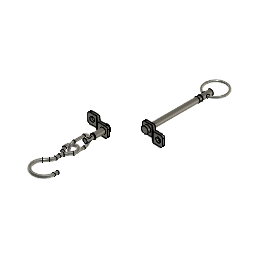
load_cell_tension_system (Autodesk Fusion 360 design; units mm, degrees)
Autodesk Fusion 360 part; units mm, degrees
note: some values were not read from the file. Chosen so that the rebuilt part matches the saved one: which face or edge a step refers to; a direction. Set by a fixed rule: which sketch regions a step uses.
sketch "Sketch1" plane through (0, 0, 0) normal (0, 0, 1) x (1, 0, 0)
  line L0 (30, -6.35) -> (-30, -6.35) construction
  line L1 (-30, -6.35) -> (-30, 6.35) construction
  line L2 (-30, 6.35) -> (30, 6.35) construction
  line L3 (30, 6.35) -> (30, -6.35) construction
  line L4 (30, -6.35) -> (-30, 6.35) construction
  line L5 (-30, -6.35) -> (30, 6.35) construction
  line L6 (-29.2721, -6.35) -> (-20, -6.35)
  line L7 (-20, -6.35) -> (-14.636, -10.8509)
  line L8 (-14.636, -10.8509) -> (-5.364, -10.8509)
  line L9 (-29.2721, -8.35) -> (-20.7279, -8.35)
  line L10 (-20.7279, -8.35) -> (-15.364, -12.8509)
  line L11 (-15.364, -12.8509) -> (-5.364, -12.8509)
  line L12 (-29.2721, -6.35) -> (-29.2721, -8.35)
  line L13 (-5.364, -10.8509) -> (-5.364, -12.8509)
  point P0 (-25, -8.35)
  point P1 (-10, -10.8509)
  dimension "d1" = 12.7
  dimension "d2" = 60
  dimension "d3" = 2
  dimension "d4" = 140
  dimension "d6" = 10
  dimension "d7" = 5
  dimension "d9" = 15
  constraint horizontal L0
  constraint perpendicular L0 L1
  constraint parallel L0 L2
  constraint parallel L1 L3
  constraint coincident L4 origin
  constraint coincident L5 origin
  constraint coincident L0 L6.start
  constraint coincident L0 L6.end
  constraint parallel L0 L8
  constraint equal L6 L8
  constraint vertical L12
  constraint vertical L13
  constraint midpoint L9 P0
  constraint midpoint L8 P1
  measures "d1" distance of L0.end L1.end
  measures "d2" distance of L0.start L0.end
  measures "d4" angle of L7 L8
  measures "d6" distance of L10.end L11.end
  measures "d7" horizontal distance of L0.end P0
  measures "d9" horizontal distance of P0 P1
extrude "Extrude1" add sketch "Sketch1" along normal mid plane 10 makes body 1
fillet "Fillet1" radius 2 4 edges at (-5.364, -11.8509, 5) (-5.364, -11.8509, -5) (-29.2721, -7.35, 5) (-29.2721, -7.35, -5) on bodies 1
sketch "Sketch2" plane through (0, -8.35, 0) normal (0, -1, 0) x (1, 0, 0)
  arc A0 (-29.2721, -3) -> (-27.2721, -5) centre (-27.2721, -3) ccw
  line L0 (-27.2721, -5) -> (-20.7279, -5)
  line L1 (-20.7279, -5) -> (-20.7279, 5)
  line L2 (-20.7279, 5) -> (-27.2721, 5)
  arc A1 (-27.2721, 5) -> (-29.2721, 3) centre (-27.2721, 3) ccw
  line L3 (-29.2721, 3) -> (-29.2721, -3)
  point P0 (-25, 0)
  point P1 (-10, 0)
hole "Hole1" at (-25, -8.35, 0) direction (0, 1, 0) diameter 4.5 depth 7 tip angle 180 bodies 1
hole "Hole2" at (-10, -8.35, 0) direction (0, -1, 0) diameter 5.5 depth 7 tip angle 180 bodies 1
mirror "Mirror1" about plane through (0, 0, 0) normal (1, 0, 0) of bodies 1 makes body 2
mirror "Mirror2" about plane through (0, 0, 0) normal (0, 1, 0) of bodies 2 makes body 3
delete_body "RemoveBody1" bodies 2
sketch "Sketch3" plane through (0, 12.8509, 0) normal (0, 1, 0) x (-1, 0, 0)
  circle A0 centre (-10, 0) radius 2.75
  arc A1 (-7.364, -5) -> (-5.364, -3) centre (-7.364, -3) ccw
  line L0 (-5.364, -3) -> (-5.364, 3)
  arc A2 (-5.364, 3) -> (-7.364, 5) centre (-7.364, 3) ccw
  line L1 (-7.364, 5) -> (-15.364, 5)
  line L2 (-15.364, 5) -> (-15.364, -5)
  line L3 (-15.364, -5) -> (-7.364, -5)
  circle A3 centre (-10, 0) radius 2.5
  dimension "d24" = 5
  constraint concentric A0 A3
  measures "d24" diameter of A3
extrude "Extrude2" add sketch "Sketch3" along normal blind 60 and the other way blind 2.1 separate body contours A3 makes body 4
sketch "Sketch4" plane through (0, 0, 0) normal (0, 0, 1) x (1, 0, 0)
  line L0 (12, 62.8509) -> (14.4908, 62.8509)
  line L1 (14.4908, 62.8509) -> (14.4908, 59.8509)
  line L2 (14.4908, 59.8509) -> (12, 59.8509)
  line L3 (12, 59.8509) -> (12, 62.8509)
  line L4 (12.5, 72.8509) -> (7.5, 72.8509)
  line L5 (10, 72.8509) -> (10, 59.2926)
  line L6 (7.5, 10.7509) -> (12.5, 10.7509)
  line L7 (12.5, 10.7509) -> (13, 10.7509)
  line L8 (10, 10.7509) -> (10, 10.2509)
  line L9 (13, 10.7509) -> (13, 10.2509)
  line L10 (13, 10.2509) -> (10, 10.2509)
  dimension "d29" = 2
  dimension "d30" = 3
  dimension "d31" = 10
  dimension "d33" = 0.5
  dimension "d35" = 0.5
  constraint horizontal L0
  constraint vertical L1
  constraint horizontal L2
  constraint vertical L3
  constraint midpoint L4 L5.start
  constraint perpendicular L4 L5
  constraint coincident L6.end L7.start
  constraint horizontal L7
  constraint midpoint L6 L8.start
  constraint vertical L8
  constraint perpendicular L7 L9
  constraint horizontal L10
  measures "d29" distance of L3 L5
  measures "d30" distance of L0.start L2.end
  measures "d31" distance of L0.start L4
  measures "d33" distance of L6.end L7.end
  measures "d35" distance of L8.end L8.start
revolve "Revolve1" cut sketch "Sketch4" angle 360 about axis through (10, 72.8509, 0) along (0, -1, 0) contours L0 L1 L2 L3 bodies 4
revolve "Revolve2" add sketch "Sketch4" angle 360 about axis through (10, 10.7509, 0) along (0, -1, 0) contours L6 L7 L8 L9 L10 bodies 4
ref_plane "WorkPlane1" through (10, 66.0717, 0) normal (-1, 0, 0) x (0, -1, 0)
sketch "Sketch5" plane through (10, 0, 0) normal (-1, 0, 0) x (0, -1, 0)
  circle A0 centre (-67.8509, 0) radius 1.5
  circle A1 centre (-67.8509, 0) radius 1
  point P0 (-72.8509, 0)
  dimension "d43" = 5
  dimension "d44" = 3
  dimension "d45" = 2
  constraint concentric A0 A1
  constraint horizontal A0.centre origin
  measures "d43" distance of A0.centre P0
  measures "d44" diameter of A0
  measures "d45" diameter of A1
extrude "Extrude3" cut sketch "Sketch5" along normal mid plane 28 contours A0 | A1 bodies 4
sketch "Sketch6" plane through (0, 0, 0) normal (0, 0, 1) x (1, 0, 0)
  circle A0 centre (10, 77.8509) radius 10
  point P0 (10, 67.8509)
  dimension "d46" = 20
  constraint coincident A0 P0
  constraint vertical A0.centre P0
  measures "d46" diameter of A0
sweep "Sweep1" add profiles "Sketch5" path "Sketch6" along A0 section 1 contours A1 separate body makes body 5
sketch "Sketch7" plane through (0, 0, 0) normal (0, 0, 1) x (1, 0, 0)
  line L0 (-7.25, -12.8509) -> (-12.75, -12.8509)
  line L1 (-10, -10.2509) -> (-10, -30.2509)
  line L2 (-10, -10.2509) -> (-7, -10.2509)
  line L3 (-7, -10.2509) -> (-7, -10.7509)
  line L4 (-7, -10.7509) -> (-7.5, -10.7509)
  line L5 (-7.5, -10.7509) -> (-7.5, -22.2509)
  line L6 (-7.5, -22.2509) -> (-8, -22.2509)
  line L7 (-8, -22.2509) -> (-8, -30.2509)
  line L8 (-8, -30.2509) -> (-10, -30.2509)
  line L9 (-7.364, -10.8509) -> (-14.636, -10.8509)
  point P0 (-10, -12.8509)
  point P1 (-10, -12.8509)
  dimension "d53" = 2.5
  dimension "d54" = 0.5
  dimension "d55" = 0.1
  dimension "d56" = 20
  dimension "d57" = 8
  dimension "d58" = 0.5
  dimension "d59" = 0.5
  constraint perpendicular L0 L1
  constraint midpoint L0 P1
  constraint coincident L1 P1
  constraint coincident P1 P0
  constraint perpendicular L1 L2
  constraint perpendicular L2 L3
  constraint perpendicular L3 L4
  constraint perpendicular L5 L6
  constraint perpendicular L0 L7
  constraint perpendicular L1 L8
  constraint vertical L5
  measures "d53" distance of L1 L5
  measures "d54" distance of L3.end L4.end
  measures "d55" distance of L4 L9
  measures "d56" distance of L1.start L1.end
  measures "d57" distance of L6.end L7.end
  measures "d58" distance of L2.end L3.end
  measures "d59" distance of L5.end L6.end
revolve "Revolve3" add sketch "Sketch7" angle 360 about axis through (-10, -10.2509, 0) along (0, -1, 0) separate body makes body 6
sketch "Sketch8" plane through (0, 0, 0) normal (0, 0, 1) x (1, 0, 0)
  circle A0 centre (-10, -26.2509) radius 1.2
  line L0 (-11.25, -26.0009) -> (-11.25, -27.0009)
  arc A1 (-11.25, -27.0009) -> (-8.75, -27.0009) centre (-10, -27.0009) ccw
  line L1 (-8.75, -27.0009) -> (-8.75, -26.0009)
  arc A2 (-8.75, -26.0009) -> (-11.25, -26.0009) centre (-10, -26.0009) ccw
  line L2 (-10, -24.7509) -> (-10, -28.2509) construction
  point P0 (-10, -12.8509)
  point P1 (-10, -30.2509)
  dimension "d62" = 2.4
  dimension "d63" = 4
  dimension "d76" = 2.5
  dimension "d77" = 3.5
  dimension "d80" = 1.5
  constraint vertical A0.centre P1
  constraint tangent L0 A1
  constraint tangent A1 L1
  constraint parallel L0 L1
  constraint tangent L1 A2
  constraint tangent L0 A2
  constraint midpoint A2 L2.start
  constraint midpoint A1 L2.end
  constraint vertical L2
  constraint vertical P1 L2.start
  measures "d62" diameter of A0
  measures "d63" distance of A0.centre P1
  measures "d76" distance of L0 L1
  measures "d77" distance of L2.start L2.end
  measures "d80" distance of A0.centre L2.start
extrude "Extrude4" cut sketch "Sketch8" along normal mid plane 6 contours A0 | L0 A1 L1 A2 bodies 6
ref_plane "WorkPlane2" through (-10, -20.2509, 0) normal (-1, 0, 0) x (0, -1, 0)
sketch "Sketch9" plane through (-10, 0, 0) normal (-1, 0, 0) x (0, -1, 0)
  line L0 (41.2509, 5) -> (31.2509, 5)
  arc A0 (31.2509, 5) -> (31.2509, -5) centre (31.2509, 0) ccw
  line L1 (31.2509, -5) -> (41.2509, -5)
  arc A1 (41.2509, -5) -> (41.2509, 5) centre (41.2509, 0) ccw
  line L2 (46.2509, 0) -> (26.2509, 0) construction
  point P0 (26.2509, 0)
  dimension "d67" = 10
  dimension "d68" = 20
  constraint tangent L0 A0
  constraint tangent A0 L1
  constraint parallel L0 L1
  constraint tangent L1 A1
  constraint tangent L0 A1
  constraint midpoint A1 L2.start
  constraint midpoint A0 P0
  constraint horizontal L2
  constraint horizontal P0 L2.end
  constraint coincident P0 L2.end
  measures "d67" distance of L0 L1
  measures "d68" distance of L2.start P0
sweep "Sweep2" add profiles "Sketch8" path "Sketch9" along A1 L0 A0 L1 section 1 contours A0 separate body makes body 7
fillet "Fillet2" radius 0.5 1 edges at (-11.8647, -22.2509, -0.7232) on bodies 6
sketch "Sketch10" plane through (-10, 0, 0) normal (-1, 0, 0) x (0, -1, 0)
  circle A0 centre (38.7509, 0) radius 1.5
  point P0 (41.2509, 0)
  dimension "d81" = 2.5
  dimension "d82" = 3
  constraint horizontal A0.centre P0
  measures "d81" horizontal distance of A0.centre P0
  measures "d82" diameter of A0
sketch "Sketch11" plane through (0, 0, 0) normal (0, 0, 1) x (1, 0, 0)
  arc A0 (-5.6699, -46.2509) -> (-14.3301, -46.2509) centre (-10, -43.7509) ccw
  line L0 (-14.3301, -46.2509) -> (-11.3301, -51.4471)
  line L1 (-5.6699, -46.2509) -> (-9.1292, -52.2426)
  line L2 (-10, -55.4926) -> (-10, -59.3851)
  line L3 (-11.5207, -63.5632) -> (-14.6756, -67.323)
  arc A1 (-14.6756, -67.323) -> (2.9834, -73.9254) centre (-7.0151, -73.7509) ccw
  arc A2 (-9.1292, -52.2426) -> (-10, -55.4926) centre (-3.5, -55.4926) ccw
  arc A3 (-11.5207, -63.5632) -> (-10, -59.3851) centre (-16.5, -59.3851) ccw
  line L4 (2.9834, -73.9254) -> (3.0706, -68.9262)
  point P0 (-10, -53.7509)
  point P1 (-10, -61.7509)
  point P2 (-10, -38.7509)
  dimension "d84" = 5
  dimension "d85" = 60
  dimension "d86" = 6
  dimension "d87" = 140
  dimension "d88" = 10
  dimension "d89" = 8
  dimension "d90" = 12
  dimension "d91" = 6.5
  dimension "d99" = 5
  dimension "d100" = 10
  dimension "d101" = 1
  constraint tangent A0 L1
  constraint tangent A0 L0
  constraint vertical L2
  constraint tangent L3 A1
  constraint coincident A0 P2
  constraint vertical A0.centre P2
  constraint vertical P0 P2
  constraint coincident P0 L1
  constraint coincident P0 L2
  constraint tangent L1 A2
  constraint tangent L2 A2
  constraint coincident P1 L2
  constraint coincident P1 L3
  constraint tangent L2 A3
  constraint tangent L3 A3
  constraint equal A2 A3
  constraint tangent A1 L4
  measures "d84" radius of A0
  measures "d85" angle of L0 L1
  measures "d86" distance of A0.end L0.end
  measures "d87" angle of L2 L3
  measures "d88" radius of A1
  measures "d89" distance of P0 P1
  measures "d90" vertical distance of P1 A1.centre
  measures "d91" radius of A2
  measures "d99" distance of A1.end L4.end
  measures "d100" distance of A0.centre P0
  measures "d101" angle of L2 L4
sweep "Sweep3" add profiles "Sketch10" path "Sketch11" along L0 A0 L1 A2 L2 A3 L3 A1 L4 section 1 separate body makes body 8
fillet "Fillet3" radius 1.5 2 edges at (-12.5413, -52.1463, -0.5424) (1.6723, -68.9018, 0.5424) on bodies 8
move_face "OffsetFaces1" offset 2 1 faces at (9.6124, 10.2509, 0.6631) on bodies 4
move_face "OffsetFaces2" offset 0.2 2 faces at (12.9963, 8.9176, -0.1495) (12.9903, 10.5842, -0.2414) on bodies 4
move_face "OffsetFaces3" offset 2 1 faces at (-10.8599, -10.2509, -0.2574) on bodies 6
move_face "OffsetFaces4" offset 0.2 1 faces at (-7.0149, -9.9176, -0.2987) on bodies 6
